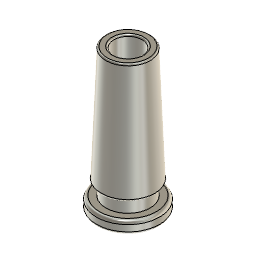
parametric_cable_gland (Autodesk Fusion 360 design; units mm, degrees)
part number: 2025-09-14-18-49-01-059
Autodesk Fusion 360 part; units mm, degrees
sketch "Sketch2" plane through (0, 0, 0) normal (1, 0, 0) x (0, 1, 0)
  line L0 (0, 0) -> (-4.5, 0) construction
  line L1 (-5, 0) -> (-9, 0)
  line L2 (-10, 1) -> (-10, 3)
  line L3 (-4.5, 0.5) -> (-4.5, 44.5)
  line L4 (-9, 4) -> (-7, 4)
  line L5 (-7, 4) -> (-7, 8)
  line L6 (-7, 8) -> (-7.719, 8)
  line L7 (-5, 45) -> (-6.5199, 45)
  line L8 (-7.0194, 44.5203) -> (-8.4684, 8.7804)
  arc A0 (-9, 4) -> (-10, 3) centre (-9, 3) ccw
  arc A1 (-10, 1) -> (-9, 0) centre (-9, 1) ccw
  arc A2 (-8.4684, 8.7804) -> (-7.719, 8) centre (-7.719, 8.75) ccw
  arc A3 (-5, 0) -> (-4.5, 0.5) centre (-5, 0.5) ccw
  arc A4 (-6.5199, 45) -> (-7.0194, 44.5203) centre (-6.5199, 44.5) ccw
  arc A5 (-4.5, 44.5) -> (-5, 45) centre (-5, 44.5) ccw
  point P0 (-10, 0)
  point P1 (-10, 4)
  point P2 (-4.5, 45)
  point P3 (-8.5, 8)
  point P4 (-7, 45)
  dimension "d6" = 4.5
  dimension "d7" = 5.5
  dimension "d8" = 4
  dimension "d9" = 45
  dimension "d10" = 2.5
  dimension "d12" = 4
  dimension "d13" = 2.5
  dimension "d15" = 1.5
  dimension "d16" = 1
  dimension "d17" = 1
  dimension "d18" = 0.75
  dimension "d19" = 0.5
  dimension "d20" = 0.5
  dimension "d21" = 0.5
  constraint coincident L0.start origin
  constraint horizontal L0
  constraint parallel L0 L1
  constraint perpendicular L1 L2
  constraint perpendicular L1 L3
  constraint perpendicular L2 L4
  constraint perpendicular L4 L5
  constraint perpendicular L2 L6
  constraint perpendicular L3 L7
  constraint coincident P1 L2
  constraint coincident P1 L4
  constraint tangent L2 A0
  constraint tangent L4 A0
  constraint coincident P0 L1
  constraint coincident P0 L2
  constraint tangent L1 A1
  constraint tangent L2 A1
  constraint coincident P3 L6
  constraint coincident P3 L8
  constraint tangent L6 A2
  constraint tangent L8 A2
  constraint coincident L0.end L3
  constraint coincident L0.end L1
  constraint tangent L3 A3
  constraint tangent L1 A3
  constraint coincident P4 L7
  constraint coincident P4 L8
  constraint tangent L7 A4
  constraint tangent L8 A4
  constraint coincident P2 L3
  constraint coincident P2 L7
  constraint tangent L3 A5
  constraint tangent L7 A5
  measures "d6" distance of L0.start L0.end
  measures "d7" distance of L0.end P0
  measures "d8" distance of P0 P1
  measures "d9" distance of L0.end P2
  measures "d10" distance of L3 L4.end
  measures "d12" distance of L4.end L5.end
  measures "d13" distance of P2 P4
  measures "d15" distance of L5.end P3
  measures "d16" radius of A0
  measures "d17" radius of A1
  measures "d18" radius of A2
  measures "d19" radius of A3
  measures "d20" radius of A4
  measures "d21" radius of A5 L0.end
revolve "Revolve1" add sketch "Sketch2" angle 360 about axis through (0, 0, 1.75) along (0, 0, 1)
equation "inner_diameter = 9 mm"
equation "flange_depth = 4 mm"
equation "flange_outer_diameter = 20 mm"
equation "length = 45 mm"
equation "grommet_outer_diameter = 14 mm"
equation "d6 = inner_diameter / 2"
equation "d7 = ( flange_outer_diameter - inner_diameter ) / 2"
equation "d8 = flange_depth"
equation "d9 = length"
equation "d10 = ( grommet_outer_diameter - inner_diameter ) / 2"
equation "grommet_height = 4 mm"
equation "d12 = grommet_height"
equation "d13 = ( grommet_outer_diameter - inner_diameter ) / 2"
equation "d15 = ( flange_outer_diameter - grommet_outer_diameter ) / 2 / 2"
equation "d18 = ( flange_outer_diameter - grommet_outer_diameter ) / 2 / 2 / 2"
